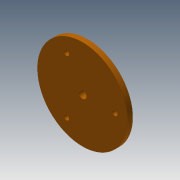
# Autodesk Inventor part: servo_paka_dolu
Saved by Autodesk Inventor 2015 (Build 190159000, 159)
## iProperties
Created: 2013-05-25
Part Number: servo_paka_dolu
Material: Generic
Document SubType Name: Modeling
Designer: idle-rug
Density: 1 g/cm^3
Appearance: Default
Author: idle-rug
Autodesk Inventor part; units mm, degrees
ref_plane "YZ Plane" through (0, 0, 0) normal (1, 0, 0) x (0, 1, 0)
ref_plane "XZ Plane" through (0, 0, 0) normal (0, 1, 0) x (-1, 0, 0)
ref_plane "XY Plane" through (0, 0, 0) normal (0, 0, 1) x (1, 0, 0)
sketch "Sketch1" plane through (0, 0, 0) normal (0, 1, 0) x (-1, 0, 0)
  circle A0 centre (0, 0) radius 17.5
  circle A1 centre (0, 0) radius 1.5
  dimension "d0" = 35
  dimension "d1" = 3
  constraints: 2 centre point, 2 coincident
  measures "d0" diameter of A0
  measures "d1" diameter of A1
extrude "Extrusion1" add sketch "Sketch1" along normal blind 2
sketch "Sketch2" plane through (0, 2, 0) normal (0, 1, 0) x (1, 0, 0)
  circle A0 centre (0, 0) radius 17.5 projected
  circle A1 centre (0, 0) radius 5
  dimension "d4" = 10
  constraints: 1 centre point, 1 coincident
  measures "d4" diameter of A1
extrude "Extrusion2" add sketch "Sketch2" along normal blind 3.8 contours A1
sketch "Sketch3" plane through (0, 5.8, 0) normal (0, 1, 0) x (1, 0, 0)
  circle A0 centre (0, 0) radius 5 projected
  circle A1 centre (0, 0) radius 3
  dimension "d7" = 6
  constraints: 1 centre point, 1 coincident
  measures "d7" diameter of A1
extrude "Extrusion3" cut sketch "Sketch3" against normal blind 3.8 contours A1
sketch "Sketch4" plane through (0, 0, 0) normal (0, -1, 0) x (1, 0, 0)
  circle A0 centre (0, 0) radius 17.5 projected
  circle A1 centre (12.5, 0) radius 1
  line L0 (0, 0) -> (-6.25, 10.8253)
  line L1 (0, 0) -> (12.5, 0) construction
  line L2 (0, 0) -> (-6.25, -10.8253)
  line L3 (0, 0) -> (12.5, 0) construction
  circle A2 centre (-6.25, 10.8253) radius 1
  circle A3 centre (-6.25, -10.8253) radius 1
  dimension "d11" = 2
  dimension "d12" = 120
  dimension "d13" = 120
  dimension "d14" = 2
  dimension "d15" = 2
  constraints: 8 end point, 3 centre point, 3 coincident, 2 equal length, 2 horizontal
  measures "d11" diameter of A1
  measures "d12" angle of L1 L0
  measures "d13" angle of L2 L3
  measures "d14" diameter of A2
  measures "d15" diameter of A3
extrude "Extrusion4" cut sketch "Sketch4" against normal blind 3.8 contours A1 | A2 | A3
body "Solid1"
